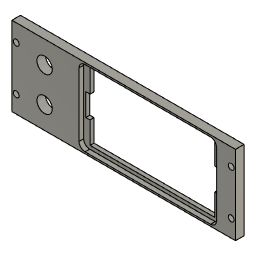
Front Panel v13 (Autodesk Fusion 360 design; units mm, degrees)
Autodesk Fusion 360 part; units mm, degrees
sketch "Sketch1" plane through (0, 0, 0) normal (0, 0, 1) x (1, 0, 0)
  line L0 (0, 0) -> (130, 0)
  line L1 (130, 0) -> (130, 5)
  line L2 (130, 5) -> (0, 5)
  line L3 (0, 5) -> (0, 0)
  dimension "d1" = 130
  dimension "d2" = 5
  constraint horizontal L0
  constraint vertical L1
  constraint horizontal L2
  constraint vertical L3
  constraint coincident L0.start L3.end
  measures "d1" distance of L0.start L0.end
  measures "d2" distance of L0.start L2.end
extrude "Extrude1" add sketch "Sketch1" along normal blind 46
sketch "Sketch2" plane through (0, 0, 0) normal (0, -1, 0) x (1, 0, 0)
  line L0 (0, 0) -> (130, 0)
  line L1 (130, 0) -> (130, 46)
  line L2 (130, 46) -> (0, 46)
  line L3 (0, 46) -> (0, 0)
  line L4 (42.5, 45) -> (115.5, 45)
  line L5 (119, 41.5) -> (119, 4.5)
  line L6 (115.5, 1) -> (42.5, 1)
  line L7 (39, 4.5) -> (39, 41.5)
  line L8 (125, 46) -> (125, 0) construction
  line L9 (5, 46) -> (5, 0) construction
  line L10 (42.75, 43) -> (115.25, 43)
  line L11 (115.25, 3) -> (42.75, 3)
  line L12 (42.75, 28.8154) -> (40.25, 28.8154)
  line L13 (40.25, 28.8154) -> (40.25, 15.8154)
  line L14 (40.25, 15.8154) -> (42.75, 15.8154)
  line L15 (115.25, 28.8154) -> (117.75, 28.8154)
  line L16 (117.75, 28.8154) -> (117.75, 15.8154)
  line L17 (117.75, 15.8154) -> (115.25, 15.8154)
  line L18 (115.25, 43) -> (115.25, 28.8154)
  line L19 (115.25, 15.8154) -> (115.25, 3)
  line L20 (42.75, 3) -> (42.75, 15.8154)
  line L21 (42.75, 28.8154) -> (42.75, 43)
  arc A0 (42.5, 45) -> (39, 41.5) centre (42.5, 41.5) ccw
  arc A1 (119, 41.5) -> (115.5, 45) centre (115.5, 41.5) ccw
  arc A2 (115.5, 1) -> (119, 4.5) centre (115.5, 4.5) ccw
  arc A3 (39, 4.5) -> (42.5, 1) centre (42.5, 4.5) ccw
  point P0 (39, 45)
  point P1 (119, 45)
  point P2 (39, 1)
  dimension "d5" = 80
  dimension "d6" = 44
  dimension "d7" = 5
  dimension "d8" = 5
  dimension "d9" = 6
  dimension "d10" = 1
  dimension "d25" = 2.5
  dimension "d26" = 13
  dimension "d28" = 13
  dimension "d35" = 3.5
  dimension "d59" = 72.5
  dimension "d60" = 40
  dimension "d62" = 2.5
  dimension "d63" = 1.25
  dimension "d64" = 2
  constraint horizontal L4
  constraint vertical L5
  constraint horizontal L6
  constraint vertical L7
  constraint coincident L2 L8.start
  constraint coincident L0 L8.end
  constraint perpendicular L0 L8
  constraint coincident L2 L9.start
  constraint coincident L0 L9.end
  constraint perpendicular L0 L9
  constraint parallel L7 L20
  constraint parallel L4 L10
  constraint parallel L6 L11
  constraint parallel L5 L18
  constraint horizontal L12
  constraint vertical L13
  constraint horizontal L14
  constraint coincident L12.start L20
  constraint horizontal L15
  constraint vertical L16
  constraint horizontal L17
  constraint collinear L18 L19
  constraint collinear L20 L21
  constraint coincident P0 L4
  constraint coincident P0 L7
  constraint tangent L4 A0
  constraint tangent L7 A0
  constraint coincident P1 L4
  constraint coincident P1 L5
  constraint tangent L4 A1
  constraint tangent L5 A1
  constraint equal A0 A1
  constraint tangent L5 A2
  constraint tangent L6 A2
  constraint equal A0 A2
  constraint coincident P2 L6
  constraint coincident P2 L7
  constraint tangent L6 A3
  constraint tangent L7 A3
  constraint equal A0 A3
  constraint horizontal L12.start L15.start
  measures "d5" distance of P0 P1
  measures "d6" distance of P0 P2
  measures "d7" distance of L1 L8
  measures "d8" distance of L3 L9
  measures "d9" distance of L5 L8
  measures "d10" distance of L2 L4
  measures "d25" distance of L12.start L12.end
  measures "d26" distance of L12.start L14.end
  measures "d28" distance of L15.start L17.end
  measures "d35" radius of A0
  measures "d59" distance of L10.start L10.end
  measures "d60" distance of L10 L11
  measures "d62" distance of L15.start L15.end
  measures "d63" distance of L7 L13
  measures "d64" distance of L4 L10
extrude "Extrude5" cut sketch "Sketch2" against normal blind 5 contours L10 L11 L12 L13 L14 L15 L16 L17 L18 L19 L20 L21
sketch "Sketch4" plane through (0, 5, 0) normal (0, 1, 0) x (-1, 0, 0)
  line L0 (-40.25, 15.8154) -> (-42.75, 15.8154)
  line L1 (-42.75, 15.8154) -> (-42.75, 3)
  line L2 (-42.75, 3) -> (-115.25, 3)
  line L3 (-115.25, 3) -> (-115.25, 15.8154)
  line L4 (-115.25, 15.8154) -> (-117.75, 15.8154)
  line L5 (-117.75, 15.8154) -> (-117.75, 28.8154)
  line L6 (-117.75, 28.8154) -> (-115.25, 28.8154)
  line L7 (-115.25, 28.8154) -> (-115.25, 43)
  line L8 (-115.25, 43) -> (-42.75, 43)
  line L9 (-42.75, 43) -> (-42.75, 28.8154)
  line L10 (-42.75, 28.8154) -> (-40.25, 28.8154)
  line L11 (-40.25, 28.8154) -> (-40.25, 15.8154)
  line L12 (-130, 0) -> (0, 0)
  line L13 (0, 0) -> (0, 46)
  line L14 (0, 46) -> (-130, 46)
  line L15 (-130, 46) -> (-130, 0)
  line L16 (-118.25, 45) -> (-39.25, 45)
  line L17 (-39.25, 45) -> (-39.25, 2)
  line L18 (-39.25, 2) -> (-118.25, 2)
  line L19 (-118.25, 2) -> (-118.25, 45)
  line L20 (-42.75, 43) -> (-115.25, 43)
  dimension "d31" = 79
  dimension "d32" = 43
  dimension "d33" = 2
  dimension "d34" = 3.5
  constraint horizontal L16
  constraint vertical L17
  constraint horizontal L18
  constraint vertical L19
  measures "d31" distance of L16.start L16.end
  measures "d32" distance of L16.start L18.end
  measures "d33" distance of L16 L20
  measures "d34" distance of L1 L17
extrude "Extrude6" cut sketch "Sketch2" against normal blind 2.7 contours L4 L5 L6 L7 A0 A1 A2 A3
sketch "Sketch5" plane through (0, 0, 0) normal (0, -1, 0) x (1, 0, 0)
  line L0 (39, 4.5) -> (39, 41.5)
  arc A0 (42.5, 45) -> (39, 41.5) centre (42.5, 41.5) ccw
  line L1 (42.5, 45) -> (115.5, 45)
  arc A1 (119, 41.5) -> (115.5, 45) centre (115.5, 41.5) ccw
  line L2 (119, 41.5) -> (119, 4.5)
  arc A2 (115.5, 1) -> (119, 4.5) centre (115.5, 4.5) ccw
  line L3 (115.5, 1) -> (42.5, 1)
  arc A3 (39, 4.5) -> (42.5, 1) centre (42.5, 4.5) ccw
  line L4 (0, 0) -> (130, 0)
  line L5 (130, 0) -> (130, 46)
  line L6 (130, 46) -> (0, 46)
  line L7 (0, 46) -> (0, 0)
  line L8 (19, 33) -> (19, 13) construction
  line L9 (5, 46) -> (5, 0) construction
  line L10 (39, 23) -> (19, 23) construction
  point P0 (19, 33)
  point P1 (19, 13)
  point P2 (19, 33)
  point P3 (19, 33)
  point P4 (19, 33)
  point P5 (19, 13)
  dimension "d40" = 20
  dimension "d41" = 20
  dimension "d42" = 5
  constraint perpendicular L6 L8
  constraint coincident L6 L9.start
  constraint coincident L4 L9.end
  constraint perpendicular L4 L9
  constraint coincident P4 P3
  constraint coincident P5 P1
  constraint midpoint L0 L10.start
  constraint midpoint L8 L10.end
  measures "d40" distance of P4 P5
  measures "d41" distance of L0 L8
  measures "d42" distance of L7 L9
hole "Hole1" at (19, 0, 33) at (19, 0, 13) direction (0, 1, 0) diameter 9 end through all
sketch "Sketch6" plane through (0, 0, 0) normal (0, -1, 0) x (1, 0, 0)
  circle A0 centre (19, 33) radius 4.5
  circle A1 centre (19, 13) radius 4.5
  line L0 (39, 4.5) -> (39, 41.5)
  arc A2 (42.5, 45) -> (39, 41.5) centre (42.5, 41.5) ccw
  line L1 (42.5, 45) -> (115.5, 45)
  arc A3 (119, 41.5) -> (115.5, 45) centre (115.5, 41.5) ccw
  line L2 (119, 41.5) -> (119, 4.5)
  arc A4 (115.5, 1) -> (119, 4.5) centre (115.5, 4.5) ccw
  line L3 (115.5, 1) -> (42.5, 1)
  arc A5 (39, 4.5) -> (42.5, 1) centre (42.5, 4.5) ccw
  line L4 (0, 0) -> (130, 0)
  line L5 (130, 0) -> (130, 46)
  line L6 (130, 46) -> (0, 46)
  line L7 (0, 46) -> (0, 0)
  line L8 (125, 46) -> (125, 0) construction
  line L9 (5, 46) -> (5, 0) construction
  point P0 (2.5, 36)
  point P1 (2.5, 10)
  point P2 (127.5, 36)
  point P3 (127.5, 10)
  dimension "d46" = 5
  dimension "d47" = 5
  dimension "d48" = 2.5
  dimension "d49" = 10
  dimension "d50" = 10
  dimension "d51" = 2.5
  dimension "d52" = 2.5
  dimension "d53" = 10
  dimension "d54" = 10
  dimension "d55" = 2.5
  constraint coincident L6 L8.start
  constraint coincident L4 L8.end
  constraint perpendicular L4 L8
  constraint coincident L6 L9.start
  constraint coincident L4 L9.end
  constraint perpendicular L4 L9
  measures "d46" distance of L5 L8
  measures "d47" distance of L7 L9
  measures "d48" distance of L9 P0
  measures "d49" distance of L6 P0
  measures "d50" distance of L4 P1
  measures "d51" distance of L9 P1
  measures "d52" distance of L8 P2
  measures "d53" distance of L6 P2
  measures "d54" distance of L4 P3
  measures "d55" distance of L8 P3
hole "Hole2" at (127.5, 0, 36) at (127.5, 0, 10) at (2.5, 0, 36) at (2.5, 0, 10) direction (0, 1, 0) diameter 3.4 depth 5 tip angle 180
